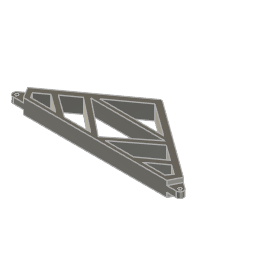
悬臂 (Autodesk Fusion 360 design; units mm, degrees)
Autodesk Fusion 360 part; units mm, degrees
note: some values were not read from the file. Chosen so that the rebuilt part matches the saved one: which face or edge a step refers to. Set by a fixed rule: which sketch regions a step uses.
sketch "草图1" plane through (0, 0, 0) normal (0, 0, 1) x (1, 0, 0)
  circle A0 centre (25.990313, 5) radius 5.009687
  circle A1 centre (244.992492, 5.015648) radius 4.992513
  line L0 (26.562836, 0.023135) -> (244.992492, 0.023135)
  line L1 (248.127038, 8.901495) -> (237.000004, 17)
  line L2 (23.127272, 9.110956) -> (135.483005, 90.742175)
  line L3 (248.127038, 8.901495) -> (88.427439, 124.930045)
  line L4 (31, 5) -> (31, 6)
  line L5 (31, 5) -> (240.000004, 5)
  line L6 (240.000004, 5) -> (107.535616, 101.241011)
  line L7 (31, 5) -> (167.226856, 103.974604)
  line L8 (31, 5) -> (199.385654, 5) construction
  line L9 (92.622426, 49.771313) -> (178.377578, 49.771313)
  line L10 (85.750287, 44.778412) -> (185.249717, 44.778412)
  line L11 (85.750287, 44.778412) -> (135.500002, 5)
  line L12 (135.500002, 5) -> (185.249717, 44.778412)
  line L13 (79.903571, 40.530524) -> (125, 5)
  line L14 (145, 5) -> (191.096433, 40.530524)
  dimension "d3" = 36
  dimension "d4" = 36
  constraint tangent A1 L0
  constraint horizontal L0
  constraint coincident A0 L4.start
  constraint tangent A0 L4
  constraint perpendicular L4 L5
  constraint horizontal L8
  constraint horizontal L9
  constraint parallel L9 L10
  constraint coincident L8 L13.end
  constraint coincident L8 L14.start
  measures "d3" angle of L5 L6
  measures "d4" angle of L7 L8
extrude "拉伸1" add sketch "草图1" along normal blind 20 contours A0 | A0 A1 L0 L5 | A0 L2 L6 L7 | L5 L7 L11 L13 | L2 L3 L6 L7 | A1 L1 L3 | L5 L6 L12 L14 | L6 L7 L9 L10 | A1 L3 L6 L7 picked at (27.428936, 6.292443) picked at (135.448743, 1.698962) picked at (77.922823, 45.434988) picked at (96.884619, 30.102979) picked at (137.743833, 85.830877) picked at (243.446608, 4.771975) picked at (173.78205, 30.102979) picked at (121.207477, 46.442712) picked at (193.257677, 45.384861)
fillet "圆角1" radius 4 1 edges at (135.483005, 90.742175, 10)
sketch "草图2" plane through (0, 0, 20) normal (0, 0, 1) x (-1, 0, 0)
  arc A0 (-137.834146, -89.033971) -> (-133.131864, -89.033971) centre (-135.483005, -85.797903) ccw
  line L0 (-133.131864, -89.033971) -> (-23.127272, -9.110956)
  arc A1 (-23.127272, -9.110956) -> (-26.562836, -0.023135) centre (-25.990313, -5) ccw
  line L1 (-26.562836, -0.023135) -> (-244.992492, -0.023135)
  arc A2 (-244.992492, -0.023135) -> (-248.127038, -8.901495) centre (-244.992492, -5.015648) ccw
  line L2 (-248.127038, -8.901495) -> (-137.834146, -89.033971)
  line L3 (-191.096433, -40.530524) -> (-240.000004, -5)
  line L4 (-240.000004, -5) -> (-145, -5)
  line L5 (-145, -5) -> (-191.096433, -40.530524)
  line L6 (-178.377578, -49.771313) -> (-92.622426, -49.771313)
  line L7 (-92.622426, -49.771313) -> (-135.500002, -80.923695)
  line L8 (-135.500002, -80.923695) -> (-178.377578, -49.771313)
  line L9 (-125, -5) -> (-31, -5)
  line L10 (-31, -5) -> (-79.903571, -40.530524)
  line L11 (-79.903571, -40.530524) -> (-125, -5)
  line L12 (-135.500002, -5) -> (-85.750287, -44.778412)
  line L13 (-85.750287, -44.778412) -> (-185.249717, -44.778412)
  line L14 (-185.249717, -44.778412) -> (-135.500002, -5)
  circle A3 centre (-25.990313, -5) radius 1.75
  circle A4 centre (-244.992492, -5.015648) radius 1.75
  dimension "d9" = 3.5
  dimension "d10" = 3.5
  constraint concentric A1 A3
  constraint concentric A2 A4
  measures "d9" diameter of A3
  measures "d10" diameter of A4
extrude "拉伸2" cut sketch "草图2" against normal blind 20 contours A3 | A4 picked at (-24.919989, -5.025698) picked at (-244.202558, -4.55958)
sketch "草图3" plane through (0, 0, 20) normal (0, 0, 1) x (-1, 0, 0)
  circle A0 centre (-244.992492, -5.015648) radius 1.75
  circle A1 centre (-25.990313, -5) radius 1.75
  arc A2 (-137.834146, -89.033971) -> (-133.131864, -89.033971) centre (-135.483005, -85.797903) ccw
  line L0 (-133.131864, -89.033971) -> (-23.127272, -9.110956)
  arc A3 (-23.127272, -9.110956) -> (-26.562836, -0.023135) centre (-25.990313, -5) ccw
  line L1 (-26.562836, -0.023135) -> (-244.992492, -0.023135)
  arc A4 (-244.992492, -0.023135) -> (-248.127038, -8.901495) centre (-244.992492, -5.015648) ccw
  line L2 (-248.127038, -8.901495) -> (-137.834146, -89.033971)
  line L3 (-191.096433, -40.530524) -> (-240.000004, -5)
  line L4 (-240.000004, -5) -> (-145, -5)
  line L5 (-145, -5) -> (-191.096433, -40.530524)
  line L6 (-178.377578, -49.771313) -> (-92.622426, -49.771313)
  line L7 (-92.622426, -49.771313) -> (-135.500002, -80.923695)
  line L8 (-135.500002, -80.923695) -> (-178.377578, -49.771313)
  line L9 (-125, -5) -> (-31, -5)
  line L10 (-31, -5) -> (-79.903571, -40.530524)
  line L11 (-79.903571, -40.530524) -> (-125, -5)
  line L12 (-135.500002, -5) -> (-85.750287, -44.778412)
  line L13 (-85.750287, -44.778412) -> (-185.249717, -44.778412)
  line L14 (-185.249717, -44.778412) -> (-135.500002, -5)
  circle A5 centre (-25.990313, -5) radius 5.009687
  circle A6 centre (-244.992492, -5.015648) radius 4.992513
  constraint concentric A1 A5
  constraint concentric A0 A6
extrude "拉伸3" cut sketch "草图3" against normal blind 6 contours A4 L2 A6 | A3 A5 picked at (-245.276332, -1.123037) picked at (-26.740513, -1.158635)
sketch "草图4" plane through (0, 0, 0) normal (0, 0, 1) x (1, 0, 0)
  line L0 (31, 5) -> (40.000001, 0)
  line L1 (31, 5) -> (31, 15)
  circle A0 centre (245.000004, 5) radius 5
  circle A1 centre (245.000004, 5) radius 1.75
  line L2 (240.000004, 5) -> (240.000004, 15)
  line L3 (240.000004, 5) -> (230, 0)
  line L4 (230, 0) -> (245.000004, 0)
  line L5 (240.000004, 15) -> (248.000004, 9)
  line L6 (40.000001, 0) -> (26, 0)
  line L7 (31, 15) -> (23, 9)
  circle A2 centre (26, 5) radius 5.05
  dimension "d15" = 3.5
  dimension "d16" = 10.1
  constraint vertical L1
  constraint concentric A0 A1
  constraint tangent A0 L2
  constraint vertical L2
  constraint tangent A0 L4
  constraint horizontal L4
  constraint tangent A0 L5
  constraint perpendicular L1 L6
  measures "d15" diameter of A1
  measures "d16" diameter of A2
extrude "拉伸4" cut sketch "草图4" along normal blind 6 contours L0 L1 A2 | L0 L6 A2 | L1 L7 A2 picked at (24.31043, 4.902158) picked at (33.807624, 2.145294) picked at (29.168129, 11.336257)
sketch "草图5" plane through (0, 0, 20) normal (0, 0, 1) x (-1, 0, 0)
  arc A0 (-247.719524, -9.197571) -> (-240.000004, -5) centre (-244.992492, -5.015648) ccw
  line L0 (-247.719524, -9.197571) -> (-137.834146, -89.033971)
  arc A1 (-137.834146, -89.033971) -> (-133.131864, -89.033971) centre (-135.483005, -85.797903) ccw
  line L1 (-133.131864, -89.033971) -> (-23.127272, -9.110956)
  arc A2 (-31, -5) -> (-23.127272, -9.110956) centre (-25.990313, -5) ccw
  line L2 (-31, -5) -> (-79.903571, -40.530524)
  line L3 (-79.903571, -40.530524) -> (-125, -5)
  line L4 (-125, -5) -> (-31, -5)
  arc A3 (-26.562836, -0.023135) -> (-31, -5) centre (-25.990313, -5) ccw
  line L5 (-26.562836, -0.023135) -> (-244.992492, -0.023135)
  arc A4 (-240.000004, -5) -> (-244.992492, -0.023135) centre (-244.992492, -5.015648) ccw
  line L6 (-240.000004, -5) -> (-145, -5)
  line L7 (-145, -5) -> (-191.096433, -40.530524)
  line L8 (-191.096433, -40.530524) -> (-240.000004, -5)
  line L9 (-178.377578, -49.771313) -> (-92.622426, -49.771313)
  line L10 (-92.622426, -49.771313) -> (-135.500002, -80.923695)
  line L11 (-135.500002, -80.923695) -> (-178.377578, -49.771313)
  line L12 (-135.500002, -5) -> (-85.750287, -44.778412)
  line L13 (-85.750287, -44.778412) -> (-185.249717, -44.778412)
  line L14 (-185.249717, -44.778412) -> (-135.500002, -5)
  line L15 (-31, -5) -> (-40.036893, -0.023135)
  line L16 (-31, -5) -> (-31, -15)
  line L17 (-31, -15) -> (-22.81545, -8.884404)
  constraint coincident A2.start L2.start
  constraint tangent A2 L16
extrude "拉伸5" cut sketch "草图5" against normal blind 6 contours A3 L5 L15 | L1 A2 L16 picked at (-33.785128, -2.154975) picked at (-29.202025, -11.229613)
sketch "草图6" plane through (0, 0, 0) normal (0, 1, 0) x (1, 0, 0)
sketch "草图7" plane through (3.657759, -5.034473, 0) normal (-0.587785, 0.809017, 0) x (-0.809017, -0.587785, 0)
  line L0 (-33.796869, 14) -> (-33.796869, 20)
  line L1 (-33.796869, 20) -> (-160.038796, 20)
  line L2 (-160.038796, 20) -> (-160.038796, 0)
  line L3 (-160.038796, 0) -> (-33.796869, 0)
  line L4 (-33.796869, 0) -> (-33.796869, 6)
  line L5 (-33.796869, 6) -> (-24.88252, 6)
  line L6 (-24.88252, 6) -> (-24.88252, 0)
  line L7 (-24.88252, 0) -> (-24.572105, 0)
  line L8 (-24.572105, 0) -> (-24.572105, 6)
  line L9 (-24.572105, 6) -> (-24.065642, 6)
  line L10 (-24.065642, 6) -> (-24.065642, 14)
  line L11 (-24.065642, 14) -> (-33.796869, 14)
  line L12 (-24.88252, 6) -> (-24.572105, 6)
extrude "拉伸6" cut sketch "草图7" against normal blind 0.4 contours L6 L7 L8 L12 picked at (-24.779049, 4)
sketch "草图8" plane through (0, 0, 0) normal (0, 0, -1) x (1, 0, 0)
  circle A0 centre (244.992492, -5.015648) radius 1.75
  line L0 (85.750287, -44.778412) -> (135.500002, -5)
  line L1 (135.500002, -5) -> (185.249717, -44.778412)
  line L2 (185.249717, -44.778412) -> (85.750287, -44.778412)
  line L3 (39.958357, -0.023135) -> (31, -5)
  line L4 (31, -5) -> (125, -5)
  line L5 (125, -5) -> (79.903571, -40.530524)
  line L6 (79.903571, -40.530524) -> (31, -5)
  line L7 (31, -5) -> (31, -14.830828)
  line L8 (31, -14.830828) -> (133.131864, -89.033971)
  arc A1 (133.131864, -89.033971) -> (137.834146, -89.033971) centre (135.483005, -85.797903) ccw
  line L9 (137.834146, -89.033971) -> (248.127038, -8.901495)
  arc A2 (248.127038, -8.901495) -> (244.992492, -0.023135) centre (244.992492, -5.015648) ccw
  line L10 (244.992492, -0.023135) -> (39.958357, -0.023135)
  line L11 (92.622426, -49.771313) -> (178.377578, -49.771313)
  line L12 (178.377578, -49.771313) -> (135.500002, -80.923695)
  line L13 (135.500002, -80.923695) -> (92.622426, -49.771313)
  line L14 (240.000004, -5) -> (191.096433, -40.530524)
  line L15 (191.096433, -40.530524) -> (145, -5)
  line L16 (145, -5) -> (240.000004, -5)
  line L17 (240.000004, -5) -> (240.000004, -15)
  line L18 (240.000004, -5) -> (232.47265, -0.023135)
  constraint perpendicular L16 L17
extrude "拉伸7" cut sketch "草图8" against normal blind 6 contours L9 A2 L10 L17 L18 picked at (239.155048, -1.68209)
sketch "草图9" plane through (0, 0, 0) normal (0, 0, 1) x (1, 0, 0)
sketch "草图10" plane through (0, 0, 20) normal (0, 0, 1) x (-1, 0, 0)
  line L0 (-135.500002, -5) -> (-85.750287, -44.778412)
  line L1 (-85.750287, -44.778412) -> (-185.249717, -44.778412)
  line L2 (-185.249717, -44.778412) -> (-135.500002, -5)
  line L3 (-178.377578, -49.771313) -> (-92.622426, -49.771313)
  line L4 (-92.622426, -49.771313) -> (-135.500002, -80.923695)
  line L5 (-135.500002, -80.923695) -> (-178.377578, -49.771313)
  line L6 (-31, -14.830828) -> (-31, -5)
  line L7 (-31, -5) -> (-79.903571, -40.530524)
  line L8 (-79.903571, -40.530524) -> (-125, -5)
  line L9 (-125, -5) -> (-31, -5)
  line L10 (-31, -5) -> (-40.036893, -0.023135)
  line L11 (-40.036893, -0.023135) -> (-244.992492, -0.023135)
  arc A0 (-240.000004, -5) -> (-244.992492, -0.023135) centre (-244.992492, -5.015648) ccw
  line L12 (-240.000004, -5) -> (-145, -5)
  line L13 (-145, -5) -> (-191.096433, -40.530524)
  line L14 (-191.096433, -40.530524) -> (-240.000004, -5)
  arc A1 (-247.719524, -9.197571) -> (-240.000004, -5) centre (-244.992492, -5.015648) ccw
  line L15 (-247.719524, -9.197571) -> (-137.834146, -89.033971)
  arc A2 (-137.834146, -89.033971) -> (-133.131864, -89.033971) centre (-135.483005, -85.797903) ccw
  line L16 (-133.131864, -89.033971) -> (-31, -14.830828)
  line L17 (-240.000004, -5) -> (-239.969198, -14.828512)
  line L18 (-240.000004, -5) -> (-240.000004, -5.063727)
  line L19 (-240.000004, -5.063727) -> (-232.543156, -0.023135)
  constraint tangent A1 L17
  constraint perpendicular L12 L18
extrude "拉伸8" cut sketch "草图10" against normal blind 6 contours L11 A0 L12 L19 | A1 L15 L17 picked at (-237.734957, -2.183762) picked at (-241.750782, -11.213251)
sketch "草图11" plane through (0, 0, 20) normal (0, 0, 1) x (-1, 0, 0)
  line L0 (-232.543156, -0.023135) -> (-239.905729, -5)
  line L1 (-239.905729, -5) -> (-145, -5)
  line L2 (-145, -5) -> (-191.096433, -40.530524)
  line L3 (-191.096433, -40.530524) -> (-240.000004, -5)
  arc A0 (-240.000004, -5.031296) -> (-240.000004, -5) centre (-244.992492, -5.015648) ccw
  line L4 (-240.000004, -5.031296) -> (-240.000004, -5.063727)
  line L5 (-240.000004, -5.063727) -> (-239.999804, -5.063592)
  line L6 (-239.999804, -5.063592) -> (-239.969198, -14.828512)
  line L7 (-239.969198, -14.828512) -> (-137.834146, -89.033971)
  arc A1 (-137.834146, -89.033971) -> (-133.131864, -89.033971) centre (-135.483005, -85.797903) ccw
  line L8 (-133.131864, -89.033971) -> (-31, -14.830828)
  line L9 (-31, -14.830828) -> (-31, -5)
  line L10 (-31, -5) -> (-79.903571, -40.530524)
  line L11 (-79.903571, -40.530524) -> (-125, -5)
  line L12 (-125, -5) -> (-31, -5)
  line L13 (-31, -5) -> (-40.036893, -0.023135)
  line L14 (-40.036893, -0.023135) -> (-232.543156, -0.023135)
  line L15 (-135.500002, -5) -> (-85.750287, -44.778412)
  line L16 (-85.750287, -44.778412) -> (-185.249717, -44.778412)
  line L17 (-185.249717, -44.778412) -> (-135.500002, -5)
  line L18 (-178.377578, -49.771313) -> (-92.622426, -49.771313)
  line L19 (-92.622426, -49.771313) -> (-135.500002, -80.923695)
  line L20 (-135.500002, -80.923695) -> (-178.377578, -49.771313)
  line L21 (-31, -14.830828) -> (-40.036893, -0.023135)
  line L22 (-232.543156, -0.023135) -> (-239.969198, -14.828512)
extrude "拉伸9" cut sketch "草图11" against normal blind 6 contours L0 L1 L22 | L12 L13 L21 | L9 L10 L21 | L3 A0 L4 L6 L22 picked at (-235.829441, -3.341045) picked at (-36.012162, -3.341045) picked at (-32.385527, -9.283587) picked at (-238.777847, -9.177901)
sketch "草图12" plane through (0, 0, 0) normal (0, 0, -1) x (1, 0, 0)
  line L0 (240.000004, -14.80613) -> (240.000004, -5)
  line L1 (240.000004, -5) -> (191.096433, -40.530524)
  line L2 (191.096433, -40.530524) -> (145, -5)
  line L3 (145, -5) -> (240.000004, -5)
  line L4 (240.000004, -5) -> (232.47265, -0.023135)
  line L5 (232.47265, -0.023135) -> (39.958357, -0.023135)
  line L6 (39.958357, -0.023135) -> (31, -5)
  line L7 (31, -5) -> (125, -5)
  line L8 (125, -5) -> (79.903571, -40.530524)
  line L9 (79.903571, -40.530524) -> (31, -5)
  line L10 (31, -5) -> (31, -14.830828)
  line L11 (31, -14.830828) -> (133.131864, -89.033971)
  arc A0 (133.131864, -89.033971) -> (137.834146, -89.033971) centre (135.483005, -85.797903) ccw
  line L12 (137.834146, -89.033971) -> (240.000004, -14.80613)
  line L13 (85.750287, -44.778412) -> (135.500002, -5)
  line L14 (135.500002, -5) -> (185.249717, -44.778412)
  line L15 (185.249717, -44.778412) -> (85.750287, -44.778412)
  line L16 (92.622426, -49.771313) -> (178.377578, -49.771313)
  line L17 (178.377578, -49.771313) -> (135.500002, -80.923695)
  line L18 (135.500002, -80.923695) -> (92.622426, -49.771313)
  line L19 (39.958357, -0.023135) -> (31, -14.830828)
  line L20 (232.47265, -0.023135) -> (240.000004, -14.80613)
extrude "拉伸10" cut sketch "草图12" against normal blind 6 contours L0 L1 L20 | L3 L4 L20 | L6 L7 L19 | L9 L10 L19 picked at (238.785071, -9.15141) picked at (235.826491, -3.341045) picked at (35.968604, -3.341045) picked at (32.377162, -9.277509)
sketch "草图13" plane through (0, 0, 20) normal (0, 0, 1) x (-1, 0, 0)
  line L0 (-236.364338, -7.641466) -> (-239.969198, -14.828512)
  line L1 (-239.969198, -14.828512) -> (-137.834146, -89.033971)
  arc A0 (-137.834146, -89.033971) -> (-133.131864, -89.033971) centre (-135.483005, -85.797903) ccw
  line L2 (-133.131864, -89.033971) -> (-31, -14.830828)
  line L3 (-31, -14.830828) -> (-35.156579, -8.019931)
  line L4 (-35.156579, -8.019931) -> (-79.903571, -40.530524)
  line L5 (-79.903571, -40.530524) -> (-125, -5)
  line L6 (-125, -5) -> (-36.999594, -5)
  line L7 (-36.999594, -5) -> (-40.036893, -0.023135)
  line L8 (-40.036893, -0.023135) -> (-232.543156, -0.023135)
  line L9 (-232.543156, -0.023135) -> (-235.039439, -5)
  line L10 (-235.039439, -5) -> (-145, -5)
  line L11 (-145, -5) -> (-191.096433, -40.530524)
  line L12 (-191.096433, -40.530524) -> (-236.364338, -7.641466)
  line L13 (-135.500002, -5) -> (-85.750287, -44.778412)
  line L14 (-85.750287, -44.778412) -> (-185.249717, -44.778412)
  line L15 (-185.249717, -44.778412) -> (-135.500002, -5)
  line L16 (-178.377578, -49.771313) -> (-92.622426, -49.771313)
  line L17 (-92.622426, -49.771313) -> (-135.500002, -80.923695)
  line L18 (-135.500002, -80.923695) -> (-178.377578, -49.771313)
  line L19 (-60.472085, -26.412723) -> (-89.980723, -4.973442)
  line L20 (-60.472085, -26.412723) -> (-23.997403, -26.412723) construction
  line L21 (-54.674629, -22.200624) -> (-78.349257, -5)
  line L22 (-54.674629, -22.200624) -> (-25.411179, -22.200624) construction
  line L23 (-211.375818, -25.796688) -> (-182.670793, -4.941266)
  line L24 (-211.375818, -25.796688) -> (-175.894455, -25.796688) construction
  line L25 (-217.651357, -21.237242) -> (-194.955016, -4.747385)
  line L26 (-217.651357, -21.237242) -> (-189.597136, -21.237242) construction
  dimension "d31" = 144
  dimension "d32" = 144
  dimension "d33" = 36
  dimension "d34" = 36
  constraint horizontal L20
  constraint horizontal L22
  constraint horizontal L24
  constraint horizontal L26
  measures "d31" angle of L19 L20
  measures "d32" angle of L21 L22
  measures "d33" angle of L23 L24
  measures "d34" angle of L25 L26
extrude "拉伸11" add sketch "草图13" against normal blind 20 contours L10 L12 L23 L25 | L4 L6 L19 L21 picked at (-196.47672, -11.932229) picked at (-76.25517, -12.137574)
sketch "草图14" plane through (0, 0, 6) normal (0, 0, -1) x (1, 0, 0)
  line L0 (23.127272, -9.110956) -> (31, -14.830828)
  line L1 (31, -14.830828) -> (35.131486, -8.0017)
  line L2 (35.131486, -8.0017) -> (31, -5)
  line L3 (31, -5) -> (36.947454, -5)
  line L4 (36.947454, -5) -> (39.958357, -0.023135)
  line L5 (39.958357, -0.023135) -> (26.562836, -0.023135)
  arc A0 (26.562836, -0.023135) -> (23.127272, -9.110956) centre (25.990313, -5) ccw
  circle A1 centre (25.990313, -5) radius 1.75
  line L6 (39.958357, -0.023135) -> (31, -14.830828)
extrude "拉伸12" add sketch "草图14" against normal blind 8 contours L2 L3 L6 picked at (34.359647, -6.000567)
sketch "草图15" plane through (0, 0, 6) normal (0, 0, -1) x (1, 0, 0)
  circle A0 centre (244.992492, -5.015648) radius 1.75
  line L0 (240.000004, -14.80613) -> (248.127038, -8.901495)
  arc A1 (248.127038, -8.901495) -> (244.992492, -0.023135) centre (244.992492, -5.015648) ccw
  line L1 (244.992492, -0.023135) -> (232.47265, -0.023135)
  line L2 (232.47265, -0.023135) -> (235.00682, -5)
  line L3 (235.00682, -5) -> (240.000004, -5)
  line L4 (240.000004, -5) -> (236.355206, -7.648101)
  line L5 (236.355206, -7.648101) -> (240.000004, -14.80613)
  line L6 (232.47265, -0.023135) -> (240.000004, -14.80613)
extrude "拉伸13" add sketch "草图15" against normal blind 8 contours L3 L4 L6 picked at (237.120676, -5.8827)
sketch "草图16" plane through (0, 0, 14) normal (0, 0, 1) x (-1, 0, 0)
  circle A0 centre (-25.990313, -5) radius 1.75
  arc A1 (-23.127272, -9.110956) -> (-26.562836, -0.023135) centre (-25.990313, -5) ccw
  line L0 (-26.562836, -0.023135) -> (-40.036893, -0.023135)
  line L1 (-40.036893, -0.023135) -> (-36.999594, -5)
  line L2 (-36.999594, -5) -> (-36.947454, -5)
  line L3 (-36.947454, -5) -> (-35.131486, -8.0017)
  line L4 (-35.131486, -8.0017) -> (-35.156579, -8.019931)
  line L5 (-35.156579, -8.019931) -> (-31, -14.830828)
  line L6 (-31, -14.830828) -> (-23.127272, -9.110956)
  circle A2 centre (-25.990313, -5) radius 2.1
  dimension "d41" = 4.2
  constraint concentric A0 A2
  measures "d41" diameter of A2
extrude "拉伸14" cut sketch "草图16" against normal blind 8 contours A2 picked at (-24.021314, -5.191271)
sketch "草图17" plane through (0, 0, 14) normal (0, 0, 1) x (-1, 0, 0)
  circle A0 centre (-244.992492, -5.015648) radius 1.75
  arc A1 (-244.992492, -0.023135) -> (-248.127038, -8.901495) centre (-244.992492, -5.015648) ccw
  line L0 (-248.127038, -8.901495) -> (-239.969198, -14.828512)
  line L1 (-239.969198, -14.828512) -> (-236.364338, -7.641466)
  line L2 (-236.364338, -7.641466) -> (-236.355206, -7.648101)
  line L3 (-236.355206, -7.648101) -> (-235.00682, -5)
  line L4 (-235.00682, -5) -> (-235.039439, -5)
  line L5 (-235.039439, -5) -> (-232.543156, -0.023135)
  line L6 (-232.543156, -0.023135) -> (-244.992492, -0.023135)
  circle A2 centre (-244.992492, -5.015648) radius 2.1
  dimension "d44" = 4.2
  constraint concentric A0 A2
  measures "d44" diameter of A2
extrude "拉伸15" cut sketch "草图17" against normal blind 8 contours A2 picked at (-245.617111, -6.892719)
sketch "草图18" plane through (0, 0, 20) normal (0, 0, 1) x (-1, 0, 0)
  line L0 (-78.349257, -5) -> (-36.999594, -5)
  line L1 (-36.999594, -5) -> (-40.036893, -0.023135)
  line L2 (-40.036893, -0.023135) -> (-232.543156, -0.023135)
  line L3 (-232.543156, -0.023135) -> (-235.039439, -5)
  line L4 (-235.039439, -5) -> (-195.30271, -5)
  line L5 (-195.30271, -5) -> (-217.651357, -21.237242)
  line L6 (-217.651357, -21.237242) -> (-236.364338, -7.641466)
  line L7 (-236.364338, -7.641466) -> (-239.969198, -14.828512)
  line L8 (-239.969198, -14.828512) -> (-137.834146, -89.033971)
  arc A0 (-137.834146, -89.033971) -> (-133.131864, -89.033971) centre (-135.483005, -85.797903) ccw
  line L9 (-133.131864, -89.033971) -> (-31, -14.830828)
  line L10 (-31, -14.830828) -> (-35.156579, -8.019931)
  line L11 (-35.156579, -8.019931) -> (-54.674629, -22.200624)
  line L12 (-54.674629, -22.200624) -> (-78.349257, -5)
  line L13 (-182.751633, -5) -> (-145, -5)
  line L14 (-145, -5) -> (-191.096433, -40.530524)
  line L15 (-191.096433, -40.530524) -> (-211.375818, -25.796688)
  line L16 (-211.375818, -25.796688) -> (-182.751633, -5)
  line L17 (-89.94417, -5) -> (-60.472085, -26.412723)
  line L18 (-60.472085, -26.412723) -> (-79.903571, -40.530524)
  line L19 (-79.903571, -40.530524) -> (-125, -5)
  line L20 (-125, -5) -> (-89.94417, -5)
  line L21 (-135.500002, -5) -> (-85.750287, -44.778412)
  line L22 (-85.750287, -44.778412) -> (-185.249717, -44.778412)
  line L23 (-185.249717, -44.778412) -> (-135.500002, -5)
  line L24 (-178.377578, -49.771313) -> (-92.622426, -49.771313)
  line L25 (-92.622426, -49.771313) -> (-135.500002, -80.923695)
  line L26 (-135.500002, -80.923695) -> (-178.377578, -49.771313)
  line L27 (-40.16327, -11.657505) -> (-45.000231, -5)
  line L28 (-35.156579, -8.019931) -> (-36.999594, -5)
  line L29 (-236.364338, -7.641466) -> (-235.039439, -5)
  line L30 (-230.178185, -12.135969) -> (-224.9936, -5)
  constraint perpendicular L11 L27
  constraint coincident L4 L30.end
  constraint perpendicular L6 L30
extrude "拉伸16" add sketch "草图18" against normal blind 20 contours L0 L11 L27 L28 | L4 L6 L29 L30 picked at (-40.721032, -7.219168) picked at (-230.070408, -7.378656)
